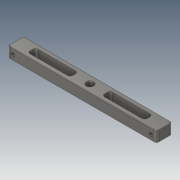
# Autodesk Inventor part: 200-60-DIFFERENTIAL-CONNECTOR-01
Saved by Autodesk Inventor 2018.2 (Build 222227000, 227)
## iProperties
Manager: feesmrt
Company: FRANC0R
Created: 2017-12-05
Part Number: 200-60-DIFFERENTIAL-CONNECTOR-01
Material: Edelstahl
Document SubType Name: Modeling
Designer: feesmrt
Density: 8 g/cm^3
Appearance: Halbpoliert
Project: Rescue Robot
Cost Center: -
Engineer: feesmrt
Authority: feesmrt
Description: Differential Bearing Connector
Stock Number: 200-60-DIFFERENTIAL-CONNECTOR-01
Mass: 288.084 g
Surface Area: 258.81 cm^2
Volume: 106.698 cm^3
Author: feesmrt
Subject: Rescue Robot
Title: Differential Bearing Connector
Revision Number: 1
Autodesk Inventor part; units mm, degrees
ref_plane "YZ Plane" through (0, 0, 0) normal (1, 0, 0) x (0, 1, 0)
ref_plane "XZ Plane" through (0, 0, 0) normal (0, 1, 0) x (-1, 0, 0)
ref_plane "XY Plane" through (0, 0, 0) normal (0, 0, 1) x (1, 0, 0)
sketch "Skizze1" plane through (0, 0, 0) normal (0, 0, 1) x (1, 0, 0)
  line L0 (-196, 0) -> (196, 0) construction
  line L1 (0, 21) -> (0, -21) construction
  line L2 (-140, -15) -> (140, -15)
  line L3 (140, -15) -> (140, 15)
  line L4 (140, 15) -> (-140, 15)
  line L5 (-140, 15) -> (-140, -15)
  line L6 (-140, -15) -> (140, 15) construction
  line L7 (140, -15) -> (-140, 15) construction
  point P0 (0, 0)
  dimension "d0" = 280
  dimension "d1" = 30
  constraints: 12 end point, 2 midpoint, 2 parallel, 1 horizontal, 1 perpendicular
  measures "d0" distance of L3.end L4.end
  measures "d1" distance of L2.end L3.end
extrude "Grundkörper" add sketch "Skizze1" along normal mid plane 20
sketch "Skizze3" plane through (0, 0, 10) normal (0, 0, 1) x (1, 0, 0)
  line L0 (0, 21) -> (0, -21) construction
  line L1 (-105, 7.5) -> (-35, 7.5)
  line L2 (-30, 2.5) -> (-30, -2.5)
  line L3 (-35, -7.5) -> (-105, -7.5)
  line L4 (-110, -2.5) -> (-110, 2.5)
  line L5 (-196, 0) -> (196, 0) construction
  line L6 (140, 15) -> (-140, 15) projected
  line L7 (0, 15) -> (-140, 15)
  line L8 (-70, 15) -> (-70, -15) construction
  line L9 (-140, -15) -> (140, -15) construction
  arc A0 (-110, -2.5) -> (-105, -7.5) centre (-105, -2.5) ccw
  arc A1 (-105, 7.5) -> (-110, 2.5) centre (-105, 2.5) ccw
  arc A2 (-30, 2.5) -> (-35, 7.5) centre (-35, 2.5) ccw
  arc A3 (-35, -7.5) -> (-30, -2.5) centre (-35, -2.5) ccw
  point P0 (0, 0)
  point P1 (-110, 7.5)
  point P2 (-30, 7.5)
  dimension "d16" = 15
  dimension "d17" = 80
  dimension "d18" = 5
  constraints: 12 end point, 8 point on circle, 8 tangent, 5 point on line, 4 centre point, 3 equal radius, 2 midpoint, 2 parallel, 1 collinear, 1 horizontal, 1 perpendicular, 1 vertical, 2 other
  measures "d16" distance between parallel lines of L3 L1
  measures "d17" distance of point (-110, 7.5) point (-30, 7.5)
  measures "d18" radius of A0
extrude "Ausschnitt_Gewichtsreduktion" cut sketch "Skizze3" against normal through all
mirror "Spiegeln_Ausschnitt_Gewichtsreduktion" about plane through (0, 0, 0) normal (1, 0, 0) of "Ausschnitt_Gewichtsreduktion"
sketch "Skizze4" plane through (0, 0, 10) normal (0, 0, 1) x (1, 0, 0)
  line L0 (0, 21) -> (0, -21) construction
  line L1 (-196, 0) -> (196, 0) construction
  point P0 (0, 0)
  point P1 (0, 0)
  constraints: 1 coincident
hole "12H7_Bohrung" at (0, 0, 10) direction (0, 0, -1) diameter 12 end through all
sketch "Skizze6" plane through (-140, -15, 10) normal (0, -1, 0) x (1, 0, 0)
  line L0 (-56, -10) -> (336, -10) projected
  line L1 (140, 4) -> (140, -24) projected
  point P0 (140, -10)
  point P1 (10.3695, -10)
  point P2 (269.6305, -10)
  dimension "d39" = 259.261
  constraints: 2 point on line, 1 symmetric about line
  measures "d39" distance of point (10.369, -10) point (269.63, -10)
hole "Bohrung3" at (-129.6305, -15, 0) at (129.6305, -15, 0) direction (0, 1, 0) diameter 6.647 end through all thread size "M8x1.25" class "6H" standard "ISO Metric profile"
fillet "Abrundung" radius 5 4 edges at (-140, 15, 0) (-140, -15, 0) (140, -15, 0) (140, 15, 0)
chamfer "Fase_Allgemein" distance 1 angle 45 16 edges at (0, -15, 10) (138.5355, -13.5355, 10) (140, 0, 10) (138.5355, 13.5355, 10) (0, 15, 10) (-138.5355, 13.5355, 10) (-140, 0, 10) (-138.5355, -13.5355, 10) (0, -15, -10) (-138.5355, -13.5355, -10) (-140, 0, -10) (-138.5355, 13.5355, -10) (0, 15, -10) (138.5355, 13.5355, -10) (140, 0, -10) (138.5355, -13.5355, -10)
chamfer "Fase_Bohrung" distance 1 angle 45 2 edges at (0, 6, 10) (0, 6, -10)
